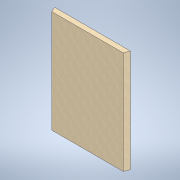
# Autodesk Inventor part: PlatteInnenzweiSeiten
Saved by Autodesk Inventor 2020.3 (Build 243373010, 373A)
## iProperties
Created: 2021-02-11
Part Number: PlatteInnenzweiSeiten
Material: Generisch
Document SubType Name: Modeling
Designer: Stefan
Density: 1 g/cm^3
Appearance: Pappel
Author: Stefan
Autodesk Inventor part; units mm, degrees
ref_plane "YZ Plane" through (0, 0, 0) normal (1, 0, 0) x (0, 1, 0)
ref_plane "XZ Plane" through (0, 0, 0) normal (0, 1, 0) x (-1, 0, 0)
ref_plane "XY Plane" through (0, 0, 0) normal (0, 0, 1) x (1, 0, 0)
sketch "Skizze1" plane through (0, 0, 0) normal (0, 0, 1) x (1, 0, 0)
  line L0 (-147.195, 0) -> (0, 0)
  line L1 (0, 0) -> (0, -200)
  line L2 (0, -200) -> (-147.195, -200)
  line L3 (-147.195, -200) -> (-147.195, 0)
  point P0 (0, 0)
  point P1 (0, 0)
  dimension "d0" = 147.195
  dimension "d1" = 200
  dimension "d2" = 0
  dimension "d3" = 0
  dimension "d4" = 0
  dimension "d5" = 0
  dimension "d6" = 0
  dimension "d7" = 200
  dimension "d8" = 147.195
  dimension "d9" = 0
  dimension "d10" = 147.195
  dimension "d11" = 200
  constraints: 8 end point, 2 parallel, 1 horizontal, 1 vertical
  measures "d0" distance between parallel lines of L1 L3
  measures "d1" distance between parallel lines of L0 L2
  measures "d2" distance from line of point (0, 0) L1
  measures "d3" distance from line of point (0, 0) L0
  measures "d4" distance from line of L0.end L1
  measures "d5" distance from line of L1.start L0
  measures "d6" distance from line of L2.start L1
  measures "d7" distance from line of L1.end L0
  measures "d8" distance from line of L0.start L1
  measures "d9" distance from line of L3.end L0
  measures "d10" distance from line of L2.end L1
  measures "d11" distance from line of L3.start L0
extrude "Extrusion1" add sketch "Skizze1" along normal blind 10
sketch "Skizze2" plane through (-147.195, -200, 0) normal (0, -1, 0) x (1, 0, 0)
  line L0 (0, 0) -> (0, 10) projected
  line L1 (0, 0) -> (4.1421, 10)
  line L2 (0, 0) -> (8.0392, 0) construction
  line L3 (0, 10) -> (147.195, 10) projected
  line L4 (0, 10) -> (4.1421, 10)
  line L5 (0, 10) -> (0, 0)
  line L6 (147.195, 0) -> (147.195, 10)
  line L7 (143.0529, 10) -> (147.195, 10)
  line L8 (147.195, 0) -> (147.195, 10) projected
  line L9 (147.195, 0) -> (143.0529, 10)
  line L10 (147.195, 0) -> (156.606, 0) construction
  point P0 (4.1421, 10)
  dimension "d14" = 67.5
  dimension "d15" = 112.5
  constraints: 16 end point, 2 horizontal, 1 collinear, 1 perpendicular, 1 vertical
  measures "d14" angle of L2 L1
  measures "d15" angle of L10 L9
extrude "Extrusion2" cut sketch "Skizze2" against normal through all
